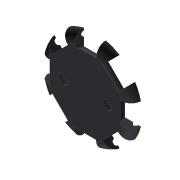
# Autodesk Inventor part: omni_wheel_cover_out_v3
Saved by Autodesk Inventor 2017 (Build 210142000, 142)
## iProperties
Created: 2018-10-27
Part Number: omni_wheel_cover_out_v3
Material: Generic
Document SubType Name: Modeling
Designer: mfans
Density: 1 g/cm^3
Appearance: Default
Author: mfans
Autodesk Inventor part; units mm, degrees
ref_plane "YZ Plane" through (0, 0, 0) normal (1, 0, 0) x (0, 1, 0)
ref_plane "XZ Plane" through (0, 0, 0) normal (0, 1, 0) x (-1, 0, 0)
ref_plane "XY Plane" through (0, 0, 0) normal (0, 0, 1) x (1, 0, 0)
sketch "Sketch1" plane through (0, 0, 0) normal (0, 1, 0) x (-1, 0, 0)
  circle A0 centre (0, 0) radius 30
  line L0 (7, 26) -> (-7, 26)
  line L1 (-7, 26) -> (-7, 19)
  line L2 (-7, 19) -> (7, 19)
  line L3 (7, 19) -> (7, 26)
  line L4 (7, 26) -> (-7, 19) construction
  line L5 (-7, 26) -> (7, 19) construction
  line L6 (7, 24.25) -> (8.7854, 24.25)
  line L7 (-7, 24.25) -> (-8.7854, 24.25)
  line L8 (9.5, 26) -> (-9.5, 26)
  arc A1 (4.5, 26) -> (7, 23.5) centre (7, 26) ccw
  arc A2 (8.7854, 24.25) -> (9.5, 26) centre (7, 26) ccw
  arc A3 (-9.5, 26) -> (-8.7854, 24.25) centre (-7, 26) ccw
  arc A4 (-7, 23.5) -> (-4.5, 26) centre (-7, 26) ccw
  point P0 (0, 22.5)
  dimension "d0" = 60
  dimension "d1" = 14
  dimension "d2" = 7
  dimension "d3" = 19
  dimension "d6" = 1.75
  dimension "d7" = 1.75
  constraints: 18 end point, 8 point on circle, 6 point on line, 5 centre point, 3 coincident, 3 horizontal, 2 midpoint, 2 parallel, 2 perpendicular
  measures "d0" diameter of A0
  measures "d1" distance of L2.end L1.end
  measures "d2" distance of L0.end L1.end
  measures "d3" distance from line of point (0, 0) L2
  measures "d6" distance between parallel lines of L0 L6
  measures "d7" distance between parallel lines of L0 L7
extrude "Extrusion1" add sketch "Sketch1" against normal blind 6 contours A0 | L3 A1 L0 | L8 A2 L6 L3 | A1 L3 L2 L1 A4 L0 | A4 L1 L0 | L1 L7 A3 L8
revolve "Revolution1" cut sketch "Sketch1" angle 360 about axis through (-7, 0, 26) along (1, 0, 0) contours L3 A1 L0 | L8 A2 L6 L3 | A1 L3 L2 L1 A4 L0 | A4 L1 L0 | L1 L7 A3 L8
sketch "Sketch2" plane through (0, -6, 0) normal (0, -1, 0) x (1, 0, 0)
  line L0 (-4.8488, 29.6056) -> (4.8488, 29.6056) projected
  arc A0 (4.8488, 29.6056) -> (-4.8488, 29.6056) centre (0, 0) ccw projected
extrude "Extrusion2" cut sketch "Sketch2" against normal blind 12
fillet "Fillet1" radius 6 1 edges at (0, -6, -30)
pattern_circular "Circular Pattern1" count 8 over 360 about axis through (0, -10, 0) along (0, 1, 0) of "Revolution1", "Extrusion2"
sketch "Sketch3" plane through (0, -6, 0) normal (0, -1, 0) x (1, 0, 0)
  point P0 (0, 0)
  point P1 (14, 0)
  point P2 (-14, 0)
  dimension "d17" = 14
  dimension "d18" = 14
  measures "d17" distance of point (0, 0) point (-14, 0)
  measures "d18" distance of point (0, 0) point (14, 0)
hole "Hole1" at (14, -6, 0) at (-14, -6, 0) direction (0, 1, 0) diameter 4 end through all
sketch "Sketch4" plane through (0, -6, 0) normal (0, -1, 0) x (1, 0, 0)
  circle A0 centre (14, 0) radius 2 projected
  circle A1 centre (-14, 0) radius 2 projected
  line L0 (-20.785, 10.8855) -> (-21.1824, 11.2829) projected
  arc A2 (-21.1824, 11.2829) -> (-22.9565, 7) centre (0, 0) ccw projected
  line L1 (-22.9565, 7) -> (-22.3944, 7) projected
  line L2 (-22.3944, 7) -> (-22.3944, -7) projected
  line L3 (-22.3944, -7) -> (-22.9565, -7) projected
  arc A3 (-22.9565, -7) -> (-21.1824, -11.2829) centre (0, 0) ccw projected
  line L4 (-21.1824, -11.2829) -> (-20.785, -10.8855) projected
  line L5 (-20.785, -10.8855) -> (-10.8855, -20.785) projected
  line L6 (-10.8855, -20.785) -> (-11.2829, -21.1824) projected
  arc A4 (-11.2829, -21.1824) -> (-7, -22.9565) centre (0, 0) ccw projected
  line L7 (-7, -22.9565) -> (-7, -22.3944) projected
  line L8 (-7, -22.3944) -> (7, -22.3944) projected
  line L9 (7, -22.3944) -> (7, -22.9565) projected
  arc A5 (7, -22.9565) -> (11.2829, -21.1824) centre (0, 0) ccw projected
  line L10 (11.2829, -21.1824) -> (10.8855, -20.785) projected
  line L11 (10.8855, -20.785) -> (20.785, -10.8855) projected
  line L12 (20.785, -10.8855) -> (21.1824, -11.2829) projected
  arc A6 (21.1824, -11.2829) -> (22.9565, -7) centre (0, 0) ccw projected
  line L13 (22.9565, -7) -> (22.3944, -7) projected
  line L14 (22.3944, -7) -> (22.3944, 7) projected
  line L15 (22.3944, 7) -> (22.9565, 7) projected
  arc A7 (22.9565, 7) -> (21.1824, 11.2829) centre (0, 0) ccw projected
  line L16 (21.1824, 11.2829) -> (20.785, 10.8855) projected
  line L17 (20.785, 10.8855) -> (10.8855, 20.785) projected
  line L18 (10.8855, 20.785) -> (11.2829, 21.1824) projected
  arc A8 (11.2829, 21.1824) -> (7, 22.9565) centre (0, 0) ccw projected
  line L19 (7, 22.9565) -> (7, 22.3944) projected
  line L20 (7, 22.3944) -> (-7, 22.3944) projected
  line L21 (-7, 22.3944) -> (-7, 22.9565) projected
  arc A9 (-7, 22.9565) -> (-11.2829, 21.1824) centre (0, 0) ccw projected
  line L22 (-11.2829, 21.1824) -> (-10.8855, 20.785) projected
  line L23 (-10.8855, 20.785) -> (-20.785, 10.8855) projected
  circle A10 centre (-14, 0) radius 2 projected
  line L24 (-14, 3.1754) -> (-11.25, 1.5877)
  line L25 (-11.25, 1.5877) -> (-11.25, -1.5877)
  line L26 (-11.25, -1.5877) -> (-14, -3.1754)
  line L27 (-14, -3.1754) -> (-16.75, -1.5877)
  line L28 (-16.75, -1.5877) -> (-16.75, 1.5877)
  line L29 (-16.75, 1.5877) -> (-14, 3.1754)
  line L30 (14, 3.1754) -> (16.75, 1.5877)
  line L31 (16.75, 1.5877) -> (16.75, -1.5877)
  line L32 (16.75, -1.5877) -> (14, -3.1754)
  line L33 (14, -3.1754) -> (11.25, -1.5877)
  line L34 (11.25, -1.5877) -> (11.25, 1.5877)
  line L35 (11.25, 1.5877) -> (14, 3.1754)
  dimension "d26" = 5.5
  dimension "d27" = 5.5
  constraints: 24 end point, 2 coincident, 26 other
  measures "d26" distance between parallel lines of L28 L25
  measures "d27" distance between parallel lines of L31 L34
extrude "Extrusion3" cut sketch "Sketch4" against normal blind 3 contours L24 L25 L26 L27 L28 L29 | L30 L31 L32 L33 L34 L35
body "Solid1"
